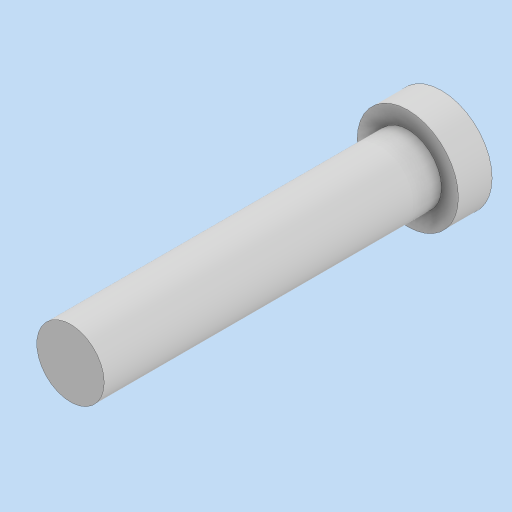
# Autodesk Inventor part: small_gripper
Saved by Autodesk Inventor 2023 (Build 270158000, 158)
## iProperties
Created: 2024-11-15
Part Number: small_gripper
Material: Generic
Document SubType Name: Modeling
Designer: ADMIN
Density: 1 g/cm^3
Appearance: Default
Author: ADMIN
Autodesk Inventor part; units mm, degrees
ref_plane "YZ Plane" through (0, 0, 0) normal (1, 0, 0) x (0, 1, 0)
ref_plane "XZ Plane" through (0, 0, 0) normal (0, 1, 0) x (-1, 0, 0)
ref_plane "XY Plane" through (0, 0, 0) normal (0, 0, 1) x (1, 0, 0)
sketch "Sketch1" plane through (0, 0, 0) normal (0, 1, 0) x (-1, 0, 0)
  line L0 (0, 0) -> (-10, 0)
  line L1 (-10, 0) -> (-10, 100)
  line L2 (-10, 100) -> (0, 100)
  line L3 (0, 100) -> (0, 0)
  line L4 (0, 0) -> (-15, 0)
  line L5 (-15, 0) -> (-15, -10)
  line L6 (-15, -10) -> (0, -10)
  line L7 (0, -10) -> (0, 0)
  dimension "d0" = 100
  dimension "d1" = 10
  dimension "d2" = 10
  dimension "d3" = 15
  constraints: 16 end point, 4 parallel, 2 horizontal, 2 perpendicular
  measures "d0" distance of L2.end L0.start
  measures "d1" distance of L1.end L2.end
  measures "d2" distance of L4.end L5.end
  measures "d3" distance of L5.end L6.end
revolve "Revolution1" add sketch "Sketch1" angle 360 about axis through (0, 0, 100) along (0, 0, -1)
body "Solid1"
